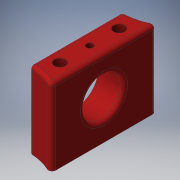
# Autodesk Inventor part: BatteryBrace
Saved by Autodesk Inventor 2016 (Build 200138000, 138)
## iProperties
Created: 2015-09-14
Part Number: BatteryBrace
Material: Generic
Document SubType Name: Modeling
Designer: lachesis
Density: 1 g/cm^3
Appearance: Default
Author: lachesis
Autodesk Inventor part; units mm, degrees
ref_plane "YZ Plane" through (0, 0, 0) normal (1, 0, 0) x (0, 1, 0)
ref_plane "XZ Plane" through (0, 0, 0) normal (0, 1, 0) x (-1, 0, 0)
ref_plane "XY Plane" through (0, 0, 0) normal (0, 0, 1) x (1, 0, 0)
sketch "Sketch1" plane through (0, 0, 0) normal (0, 1, 0) x (-1, 0, 0)
  line L0 (-4.7371, 18.5916) -> (-4.7371, -18.5916)
  line L1 (4.8895, -15.875) -> (4.8895, 15.875)
  circle A0 centre (4.8895, -34.29) radius 18.415
  circle A1 centre (4.8895, 34.29) radius 18.415
  point P0 (0, 0)
  point P1 (4.8895, 0)
  dimension "d3" = 31.75
  dimension "d10" = 36.83
  dimension "d11" = 9.6266
  dimension "d12" = 4.8895
  dimension "d13" = 0
  dimension "d14" = 0
  dimension "d15" = 16.6109
  constraints: 4 end point, 4 point on circle, 2 centre point, 1 equal radius, 1 horizontal alignment, 1 midpoint, 1 parallel, 1 vertical
  measures "d10" diameter of A1
  measures "d11" distance between parallel lines of L1 L0
  measures "d12" distance from line of point (0, 0) L1
  measures "d13" distance from line of A1.centre L1
  measures "d14" distance from line of A0.centre L1
  measures "d15" distance of point (0, 0) L1.start
extrude "Extrusion1" add sketch "Sketch1" along normal blind 26.162 contours A1 L1 A0 L0
sketch "Sketch2" plane through (4.7371, 0, 18.5916) normal (1, 0, 0) x (0, 0, -1)
  circle A0 centre (18.5916, 13.081) radius 6.731
  line L0 (0, 26.162) -> (37.1831, 26.162) projected
  line L1 (0, 0) -> (0, 26.162) projected
  point P0 (18.5916, 0)
  point P1 (18.5916, 26.162)
  point P2 (0, 13.081)
  dimension "d18" = 6.35
  constraints: 2 midpoint, 1 centre point, 1 horizontal alignment, 1 vertical alignment
  measures "d18" distance edge to line of A0 L0
extrude "Extrusion2" cut sketch "Sketch2" against normal through all
fillet "Fillet1" radius 1.27 10 edges at (4.7371, 13.081, 6.731) (-4.8895, 13.081, 6.731) (4.7371, 26.162, 0) (4.7371, 13.081, -18.5916) (4.7371, 13.081, 18.5916) (-4.8895, 13.081, 15.875) (0.1118, 26.162, 16.5671) (0.1118, 26.162, -16.5671) (-4.8895, 26.162, 0) (-4.8895, 13.081, -15.875)
sketch "Sketch3" plane through (0, 26.162, 0) normal (0, 1, 0) x (1, 0, 0)
  arc A0 (2.928, -17.6167) -> (4.7371, -16.4668) centre (3.4671, -16.4668) ccw projected
  arc A1 (4.7371, 16.4668) -> (2.928, 17.6167) centre (3.4671, 16.4668) ccw projected
  line L0 (-4.8895, 14.646) -> (-4.8895, -14.646) projected
  point P0 (0, 0)
  point P1 (-0.1905, -10.1168)
  point P2 (-0.1905, 10.1168)
  dimension "d22" = 6.35
  dimension "d23" = 6.35
  dimension "d38" = 4.699
  constraints: 1 vertical alignment
  measures "d22" vertical distance of A0.centre point (-0.191, -10.117)
  measures "d23" vertical distance of A1.centre point (-0.191, 10.117)
  measures "d38" distance from line of L0 point (-0.191, -10.117)
hole "Hole1" at (-0.1905, 26.162, 10.1168) at (-0.1905, 26.162, -10.1168) direction (0, -1, 0) diameter 3.81 end through all
sketch "Sketch4" plane through (0, 26.162, 0) normal (0, 1, 0) x (1, 0, 0)
  circle A0 centre (-0.1905, -10.1168) radius 1.905 projected
  circle A1 centre (-0.1905, 10.1168) radius 1.905 projected
  arc A2 (-3.6195, 14.646) -> (3.4671, 16.4668) centre (-4.8895, 34.29) ccw projected
  line L0 (-3.6195, -14.646) -> (-3.6195, 14.646) projected
  arc A3 (3.4671, -16.4668) -> (-3.6195, -14.646) centre (-4.8895, -34.29) ccw projected
  line L1 (3.4671, 16.4668) -> (3.4671, -16.4668) projected
  point P0 (0, 0)
  point P1 (-0.1905, 0)
  constraints: 1 horizontal alignment, 1 vertical alignment
hole "Hole2" at (-0.1905, 26.162, 0) direction (0, -1, 0) diameter 2.2606 depth 6.604
equation "\"d23\" = d22"
body "Solid1"
